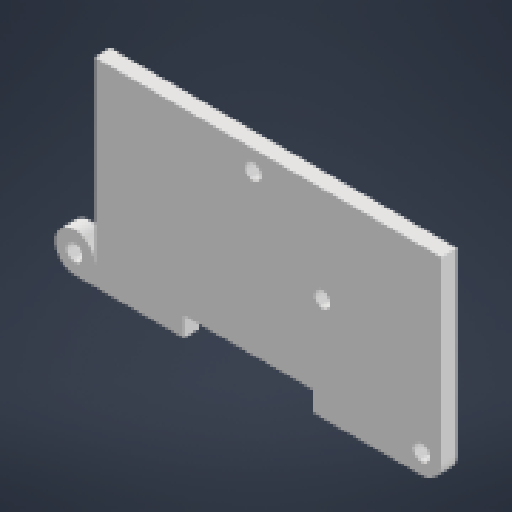
# Autodesk Inventor part: крышка захвата
Saved by Autodesk Inventor 2025 (Build 290162000, 162)
## iProperties
Created: 2025-02-22
Part Number: крышка захвата
Material: Типовые
Document SubType Name: Modeling
Designer: Phantom
Density: 1 g/cm^3
Appearance: По умолчанию
Author: Phantom
Autodesk Inventor part; units mm, degrees
ref_plane "YZ Plane" through (0, 0, 0) normal (1, 0, 0) x (0, 1, 0)
ref_plane "XZ Plane" through (0, 0, 0) normal (0, 1, 0) x (-1, 0, 0)
ref_plane "XY Plane" through (0, 0, 0) normal (0, 0, 1) x (1, 0, 0)
sketch "Эскиз1" plane through (0, 0, 0) normal (0, 0, 1) x (1, 0, 0)
  line L0 (27.5467, -7.6681) -> (1.5467, -7.6681)
  line L1 (-6.4533, -7.6681) -> (-34.4903, -7.6681)
  line L2 (-34.4903, -7.6681) -> (-6.4533, -7.6681)
  line L3 (1.5467, -7.6681) -> (27.5467, -7.6681)
  line L4 (27.5467, -7.6681) -> (27.5467, 28.4819)
  line L5 (27.5467, 28.4819) -> (-2.4533, 28.4819)
  line L6 (-2.4533, 28.4819) -> (-34.4903, 28.4819)
  line L7 (-34.4903, 28.4819) -> (-34.4903, -7.6681)
  line L8 (-34.4903, 13.2319) -> (-34.4903, 5.0319)
  line L9 (-34.4903, 3.2319) -> (-34.4903, -7.6681)
  circle A0 centre (11.5467, 9.1319) radius 1.575
  circle A1 centre (-2.4533, 24.4819) radius 1.6
  line L10 (-6.4533, -7.6681) -> (1.5467, -7.6681)
  line L11 (-16.4718, -11.6681) -> (-16.4718, -18.4681) projected
  line L12 (9.5282, -11.6681) -> (9.5282, -18.4681) projected
  line L13 (-16.4718, -18.4681) -> (9.5282, -18.4681) projected
  circle A2 centre (-38.4903, -7.6681) radius 1.6 projected
  circle A3 centre (31.5467, -7.6681) radius 1.6 projected
  arc A4 (31.5467, -11.6681) -> (27.5467, -7.6681) centre (31.5467, -7.6681) ccw projected
  line L14 (27.5467, -7.6681) -> (9.5282, -7.6681) projected
  arc A5 (-34.4903, -7.6681) -> (-38.4718, -11.6681) centre (-38.4903, -7.6681) ccw projected
  arc A6 (-38.4718, -11.6681) -> (-38.4533, -11.6681) centre (-38.4533, -7.6681) ccw projected
  line L15 (-38.4533, -11.6681) -> (-34.4903, -11.6681) projected
  arc A7 (-19.6718, -21.6681) -> (-34.4903, -11.6681) centre (-35.1698, -28.6545) ccw projected
  line L16 (12.7282, -21.6681) -> (-19.6718, -21.6681) projected
  arc A8 (27.5467, -11.6681) -> (12.7282, -21.6681) centre (28.2263, -28.6545) ccw projected
  line L17 (27.5467, -11.6681) -> (31.5467, -11.6681) projected
  arc A9 (35.5467, -7.6681) -> (27.5467, -7.6681) centre (31.5467, -7.6681) ccw projected
  line L18 (35.5467, 28.4819) -> (35.5467, -7.6681) projected
  line L19 (35.5467, 28.4819) -> (-2.4533, 28.4819) projected
  circle A10 centre (-2.4533, 24.4819) radius 4 projected
  line L20 (-2.4533, 28.4819) -> (-42.4533, 28.4819) projected
  line L21 (-42.4533, -7.1253) -> (-42.4533, 28.4819) projected
  arc A11 (-34.4903, -7.6681) -> (-42.4533, -7.1253) centre (-38.4903, -7.6681) ccw projected
  line L22 (-34.4903, -7.6681) -> (27.5467, -7.6681) projected
  arc A12 (-34.4903, 3.2319) -> (-34.4903, 5.0319) centre (-30.4903, 4.1319) ccw projected
  line L23 (-34.4903, 3.2319) -> (-34.4903, 5.0319) projected
  line L24 (-34.4903, 13.2319) -> (-34.4903, 15.0319) projected
  arc A13 (-34.4903, 13.2319) -> (-34.4903, 15.0319) centre (-30.4903, 14.1319) ccw projected
  circle A14 centre (17.5097, 4.1319) radius 4.1 projected
  circle A15 centre (-16.4533, 9.1319) radius 7 projected
  circle A16 centre (11.5467, 9.1319) radius 3.5 projected
  circle A17 centre (17.5097, 14.1319) radius 4.1 projected
  line L25 (35.5467, 28.4819) -> (27.5467, 28.4819)
  line L26 (27.5467, 28.4819) -> (27.5467, -11.6681)
  line L27 (27.5467, -11.6681) -> (35.5467, -11.6681)
  line L28 (35.5467, -11.6681) -> (35.5467, 28.4819)
  line L29 (-42.4533, 28.4819) -> (-34.4903, 28.4819)
  line L30 (-34.4903, 28.4819) -> (-34.4903, -11.6681)
  line L31 (-34.4903, -11.6681) -> (-42.4533, -11.6681)
  line L32 (-42.4533, -11.6681) -> (-42.4533, 28.4819)
  line L33 (27.5467, -11.6681) -> (-34.4903, -11.6681)
  line L34 (-34.4903, -11.6681) -> (-34.4903, -7.6681)
  line L35 (-34.4903, -7.6681) -> (27.5467, -7.6681)
  line L36 (27.5467, -7.6681) -> (27.5467, -11.6681)
  line L37 (9.5282, -7.6681) -> (9.5282, -11.6681) projected
  line L38 (-16.4718, -11.6681) -> (-16.4718, -7.6681) projected
  line L39 (-16.4718, -7.6681) -> (-34.4903, -7.6681) projected
  point P0 (0, 0)
  point P1 (-2.4533, -2.0181)
  point P2 (1.5467, -7.6681)
  point P3 (-42.4533, -8.2109)
  constraints: 46 end point, 6 parallel, 4 horizontal, 3 perpendicular, 2 centre point, 1 vertical alignment
extrude "Выдавливание1" add sketch "Эскиз1" along normal blind 3.2 contours L26 L33 L37 L0 | A10 | L0 L10 L1 L7 A12 A13 L6 L5 L4 | L4 L19 L18 A4 | A4 L17 L26 | L37 L33 L38 L1 L10 L0 | L33 L30 L1 L38 | L7 A5 L21 L20 | L15 A6 A5 L32 L30 | A13 L7 | L32 A5 | L7 A12 | A14 | A15 | A16 | A17
sketch "Эскиз2" plane through (0, 0, 3.2) normal (0, 0, 1) x (1, 0, 0)
  line L0 (-16.4718, -7.6681) -> (-13.4718, -7.6681) projected
  line L1 (6.5282, -7.6681) -> (9.5282, -7.6681) projected
  line L2 (-38.4533, -11.6681) -> (31.5467, -11.6681) projected
  line L3 (9.5282, -11.6681) -> (-16.4718, -11.6681)
  line L4 (-16.4718, -11.6681) -> (-16.4718, -7.6681)
  line L5 (-16.4718, -7.6681) -> (9.5282, -7.6681)
  line L6 (9.5282, -7.6681) -> (9.5282, -11.6681)
  line L7 (-16.4718, -7.6681) -> (9.5282, -7.6681)
  line L8 (9.5282, -7.6681) -> (9.5282, 2.3319)
  line L9 (9.5282, 2.3319) -> (-16.4718, 2.3319)
  line L10 (-16.4718, 2.3319) -> (-16.4718, -7.6681)
  point P0 (0, 0)
  point P1 (-16.4718, -11.6681)
  dimension "d4" = 26
  dimension "d5" = 10
  constraints: 16 end point, 4 parallel, 2 horizontal, 2 perpendicular, 1 point on line
  measures "d4" distance of L9.end L8.end
  measures "d5" distance of L8.end L7.end
extrude "Выдавливание2" cut sketch "Эскиз2" against normal blind 3.2
fillet "Сопряжение1" radius 2 2 edges at (9.5282, 2.3319, 1.6) (-16.4718, 2.3319, 1.6)
